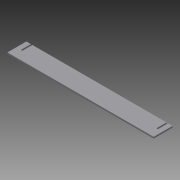
# Autodesk Inventor part: brace
Saved by Autodesk Inventor 2017 (Build 210142000, 142)
## iProperties
Created: 2019-02-02
Part Number: brace
Material: Generic
Document SubType Name: Modeling
Designer: ari
Density: 1 g/cm^3
Appearance: Default
Author: ari
Autodesk Inventor part; units mm, degrees
ref_plane "YZ Plane" through (0, 0, 0) normal (1, 0, 0) x (0, 1, 0)
ref_plane "XZ Plane" through (0, 0, 0) normal (0, 1, 0) x (-1, 0, 0)
ref_plane "XY Plane" through (0, 0, 0) normal (0, 0, 1) x (1, 0, 0)
sketch "Sketch1" plane through (0, 0, 0) normal (0, 0, 1) x (1, 0, 0)
  line L0 (0, 0) -> (385.2, 0)
  line L1 (385.2, 0) -> (385.2, 50)
  line L2 (385.2, 50) -> (373.2, 50)
  line L3 (0, 50) -> (0, 0)
  line L4 (15.85, 50) -> (15.85, 25)
  line L5 (15.85, 25) -> (12, 25)
  line L6 (12, 25) -> (12, 50)
  line L7 (192.6, 50) -> (192.6, 0) construction
  line L8 (369.35, 50) -> (369.35, 25)
  line L9 (369.35, 25) -> (373.2, 25)
  line L10 (373.2, 25) -> (373.2, 50)
  line L11 (12, 50) -> (0, 50)
  line L12 (369.35, 50) -> (15.85, 50)
  line L13 (0, 25) -> (12, 25) construction
  arc A0 (12, 25) -> (15.85, 25) centre (13.925, 25) ccw
  arc A1 (369.35, 25) -> (373.2, 25) centre (371.275, 25) ccw
  dimension "d0" = 3.85
  dimension "d1" = 50
  dimension "d2" = 361.2
  dimension "d3" = 12
  constraints: 28 end point, 6 parallel, 5 midpoint, 5 perpendicular, 4 collinear, 4 point on circle, 2 centre point, 1 horizontal, 1 other
  measures "d0" distance of L4.end L5.end
  measures "d1" distance of L3.start L0.start
  measures "d2" distance between parallel lines of L10 L6
  measures "d3" distance of L6.end L3.start
extrude "Extrusion1" add sketch "Sketch1" along normal blind 3.8 contours L3 L11 L6 A0 L4 L12 L8 A1 L10 L2 L1 L0
equation "\"d0\" = d + u"
equation "\"d4\" = d"
equation "\"d\" = 3.8"
equation "\"u\" = 0.05"
body "Solid1"
